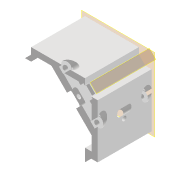
# Autodesk Inventor part: 20_Cube_Insert_Kinematic_Mirror_45_pro_v3
Saved by Autodesk Inventor 2022 (Build 260153000, 153)
## iProperties
Created: 2022-01-05
Part Number: 20_Cube_Insert_Kinematic_Mirror_45_pro_v3
Material: Generisch
Document SubType Name: Modeling
Designer: diederichbenedict
Density: 1 g/cm^3
Appearance: Vorgabe
Author: diederichbenedict
Autodesk Inventor part; units mm, degrees
ref_plane "YZ Plane" through (0, 0, 0) normal (1, 0, 0) x (0, 1, 0)
ref_plane "XZ Plane" through (0, 0, 0) normal (0, 1, 0) x (-1, 0, 0)
ref_plane "XY Plane" through (0, 0, 0) normal (0, 0, 1) x (1, 0, 0)
ref_plane "Arbeitsebene1" through (0, 0, 0) normal (0, 0, 1) x (1, 0, 0)
sketch "Skizze1" plane through (0, 0, 0) normal (0, 0, 1) x (1, 0, 0)
  arc A0 (24.85, 22.85) -> (22.85, 24.85) centre (22.85, 22.85) ccw projected
  line L0 (22.85, 24.85) -> (-16.97, 24.85) projected
  line L1 (-16.97, 24.85) -> (-16.97, 21.15) projected
  line L2 (-16.97, 21.15) -> (16.97, 21.15) projected
  line L3 (16.97, 16.97) -> (16.97, 21.15) projected
  line L4 (21.15, 16.97) -> (16.97, 16.97) projected
  line L5 (21.15, 16.97) -> (21.15, -16.97) projected
  line L6 (21.15, -16.97) -> (24.85, -16.97) projected
  line L7 (24.85, -16.97) -> (24.85, 22.85) projected
  line L8 (23.75, 23.25) -> (23.75, 18.15) projected
  arc A1 (23.25, 17.65) -> (23.75, 18.15) centre (23.25, 18.15) ccw projected
  line L9 (23.25, 17.65) -> (20.8937, 17.65) projected
  arc A2 (20.5239, 17.8134) -> (20.8937, 17.65) centre (20.8937, 18.15) ccw projected
  line L10 (20.5239, 17.8134) -> (17.7803, 20.8273) projected
  arc A3 (17.65, 21.1639) -> (17.7803, 20.8273) centre (18.15, 21.1639) ccw projected
  line L11 (17.65, 21.1639) -> (17.65, 23.25) projected
  arc A4 (18.15, 23.75) -> (17.65, 23.25) centre (18.15, 23.25) ccw projected
  line L12 (18.15, 23.75) -> (23.25, 23.75) projected
  arc A5 (23.75, 23.25) -> (23.25, 23.75) centre (23.25, 23.25) ccw projected
  line L13 (-16.87, 24.85) -> (16.87, 24.85)
  line L14 (16.87, 24.85) -> (16.87, 21.85)
  line L15 (16.87, 21.85) -> (-16.87, 21.85)
  line L16 (-16.87, 21.85) -> (-16.87, 24.85)
  line L17 (34.79, 34.79) -> (-34.79, -34.79)
  line L18 (16.87, 21.85) -> (16.87, 16.87)
  line L19 (12.87, 21.85) -> (12.87, 12.87)
  line L20 (16.87, 16.87) -> (12.87, 12.87)
  line L21 (-16.97, 21.15) -> (-16.97, 16.97) projected
  line L22 (16.97, 16.97) -> (-16.97, 16.97) projected
  line L23 (16.97, 21.15) -> (16.97, 16.97) projected
  line L24 (-16.97, 21.15) -> (16.97, 21.15) projected
  line L25 (-16.97, 16.97) -> (-16.97, 20.75) projected
  line L26 (-20.75, 16.97) -> (-16.97, 20.75) projected
  line L27 (-20.75, 16.97) -> (-16.97, 16.97) projected
  line L28 (-16.87, 21.85) -> (-12.87, 21.85)
  line L29 (-12.87, 21.85) -> (-12.87, 16.97)
  line L30 (-12.87, 16.97) -> (-16.87, 16.97)
  line L31 (-16.87, 16.97) -> (-16.87, 21.85)
  line L32 (-16.87, 20.7793) -> (-20.6793, 16.97)
  line L33 (-20.6793, 16.97) -> (-16.87, 16.97)
  line L34 (-4.8794, 21.85) -> (21.15, -4.1794)
  line L35 (-7.0711, 15.5563) -> (3.471, 5.0143) projected
  line L36 (21.15, 2.8916) -> (2.1916, 21.85)
  line L37 (12.0208, 12.0208) -> (8.4853, 8.4853)
  line L38 (20.75, 16.97) -> (16.97, 20.75) projected
  line L39 (16.97, 20.6793) -> (20.6793, 16.97)
  point P0 (0, 0)
  point P1 (-12.87, 21.15)
  point P2 (12.87, 21.15)
  point P3 (2.8916, 21.15)
  point P4 (-4.1794, 21.15)
  point P5 (12.87, 16.97)
  point P6 (16.87, 21.15)
  dimension "d0" = 0.1
  dimension "d1" = 0.1
  dimension "d2" = 3
  dimension "d3" = 4
  dimension "d6" = 4
  dimension "d8" = 0
  dimension "d9" = 0.05
  dimension "d10" = 6
  dimension "d11" = 5
  dimension "d12" = 0.05
  constraints: 36 end point, 16 point on line, 8 parallel, 2 horizontal, 2 perpendicular, 1 collinear, 1 vertical, 3 other
  measures "d0" distance between parallel lines of L16 L1
  measures "d1" distance between parallel lines of L14 L3
  measures "d2" distance between parallel lines of L0 L15
  measures "d3" distance between parallel lines of L18 L19
  measures "d6" distance of L29.end L30.end
  measures "d8" distance between parallel lines of L30 L22
  measures "d9" distance between parallel lines of L26 L32
  measures "d10" distance between parallel lines of L35 L34
  measures "d11" distance between parallel lines of L36 L34
  measures "d12" distance between parallel lines of L39 L38
extrude "Extrusion1" add sketch "Skizze1" along normal blind 33.8 contours L14 L15 L16 L0 | L18 L2 L19 L15 | L34 L22 L36 L17 | L15 L29 L2 L31 | L19 L2 L36 L15 | L18 L22 L19 L2 | L2 L3 L22 L18 | L39 L4 L17 | L17 L3 L39 | L34 L2 L36 L22 | L15 L34 L2 L29 | L2 L29 L22 L31 | L36 L2 L34 L15 | L31 L22 L21 L32 | L21 L27 L32
mirror "Spiegeln1" about plane through (8.4853, 8.4853, 0) normal (0.7071, -0.7071, 0) of "Extrusion1"
chamfer "Fase1" distance 4 angle 45 3 edges at (12.87, 16.97, 16.9) (16.97, 12.87, 16.9) (-12.87, 16.97, 16.9)
ref_plane "Arbeitsebene2" through (21.9197, 25.629, 0) normal (0.7071, 0.7071, 0) x (-0.7071, 0.7071, 0)
sketch "Skizze2" plane through (21.9197, 25.629, 0) normal (0.7071, 0.7071, 0) x (-0.7071, 0.7071, 0)
  line L0 (-16.6229, 20.13) -> (-16.6229, 14.13) projected
  arc A0 (-19.6229, 14.13) -> (-16.6229, 14.13) centre (-18.1229, 14.13) ccw projected
  line L1 (-19.6229, 14.13) -> (-19.6229, 20.13) projected
  arc A1 (-16.6229, 20.13) -> (-19.6229, 20.13) centre (-18.1229, 20.13) ccw projected
  line L2 (0.3771, 31.21) -> (-5.6229, 31.21) projected
  arc A2 (-5.6229, 34.21) -> (-5.6229, 31.21) centre (-5.6229, 32.71) ccw projected
  line L3 (-5.6229, 34.21) -> (0.3771, 34.21) projected
  arc A3 (0.3771, 31.21) -> (0.3771, 34.21) centre (0.3771, 32.71) ccw projected
  circle A4 centre (-16.6229, 31.13) radius 3.25 projected
  circle A5 centre (-2.6229, 17.13) radius 3.25 projected
  circle A6 centre (11.3771, 31.13) radius 3.25 projected
  circle A7 centre (-16.6229, 3.13) radius 3.25 projected
  line L4 (14.3357, 42.03) -> (-19.6229, 42.03) projected
  line L5 (-19.6229, 42.03) -> (-19.6229, 38.4552) projected
  line L6 (-19.6229, 38.4552) -> (-23.9481, 34.13) projected
  line L7 (-23.9481, 34.13) -> (-27.5229, 34.13) projected
  line L8 (-27.5229, 34.13) -> (-27.5229, 0.13) projected
  line L9 (-27.5229, 0.13) -> (-23.9481, 0.13) projected
  line L10 (-23.9481, 0.13) -> (-19.6229, -4.1952) projected
  line L11 (-19.6229, -4.1952) -> (-19.6229, -7.77) projected
  line L12 (-19.6229, -7.77) -> (14.3771, -7.77) projected
  line L13 (14.3771, -7.77) -> (14.3771, -4.1952) projected
  line L14 (14.3771, -4.1952) -> (18.7023, 0.13) projected
  line L15 (18.7023, 0.13) -> (22.2771, 0.13) projected
  line L16 (22.2771, 0.13) -> (22.2771, 34.13) projected
  line L17 (22.2771, 34.13) -> (18.7023, 34.13) projected
  line L18 (18.7023, 34.13) -> (14.3357, 38.4966) projected
  line L19 (14.3357, 38.4966) -> (14.3357, 42.03) projected
  point P0 (-2.6229, 0)
hole "Bohrung1" at (13.8749, 33.6739, 31.13) at (33.6739, 13.8749, 31.13) at (33.6739, 13.8749, 3.13) direction (-0.7071, -0.7071, 0) diameter 2.8 depth 30 tip angle 118 counterbore diameter 6.5 counterbore depth 17
sketch "Skizze3" plane through (16.97, 20.6793, 0) normal (0.7071, 0.7071, 0) x (-0.7071, 0.7071, 0)
  line L0 (-16.6229, 20.13) -> (-16.6229, 14.13) projected
  arc A0 (-19.6229, 14.13) -> (-16.6229, 14.13) centre (-18.1229, 14.13) ccw projected
  line L1 (-19.6229, 14.13) -> (-19.6229, 20.13) projected
  arc A1 (-16.6229, 20.13) -> (-19.6229, 20.13) centre (-18.1229, 20.13) ccw projected
  line L2 (0.3771, 31.21) -> (-5.6229, 31.21) projected
  arc A2 (-5.6229, 34.21) -> (-5.6229, 31.21) centre (-5.6229, 32.71) ccw projected
  line L3 (-5.6229, 34.21) -> (0.3771, 34.21) projected
  arc A3 (0.3771, 31.21) -> (0.3771, 34.21) centre (0.3771, 32.71) ccw projected
  circle A4 centre (-16.6229, 31.13) radius 3.25 projected
  circle A5 centre (-2.6229, 17.13) radius 3.25 projected
  circle A6 centre (11.3771, 31.13) radius 3.25 projected
  circle A7 centre (-16.6229, 3.13) radius 3.25 projected
  line L4 (14.3357, 42.03) -> (-19.6229, 42.03) projected
  line L5 (-19.6229, 42.03) -> (-19.6229, 38.4552) projected
  line L6 (-19.6229, 38.4552) -> (-23.9481, 34.13) projected
  line L7 (-23.9481, 34.13) -> (-27.5229, 34.13) projected
  line L8 (-27.5229, 34.13) -> (-27.5229, 0.13) projected
  line L9 (-27.5229, 0.13) -> (-23.9481, 0.13) projected
  line L10 (-23.9481, 0.13) -> (-19.6229, -4.1952) projected
  line L11 (-19.6229, -4.1952) -> (-19.6229, -7.77) projected
  line L12 (-19.6229, -7.77) -> (14.3771, -7.77) projected
  line L13 (14.3771, -7.77) -> (14.3771, -4.1952) projected
  line L14 (14.3771, -4.1952) -> (18.7023, 0.13) projected
  line L15 (18.7023, 0.13) -> (22.2771, 0.13) projected
  line L16 (22.2771, 0.13) -> (22.2771, 34.13) projected
  line L17 (22.2771, 34.13) -> (18.7023, 34.13) projected
  line L18 (18.7023, 34.13) -> (14.3357, 38.4966) projected
  line L19 (14.3357, 38.4966) -> (14.3357, 42.03) projected
  point P0 (-2.6229, 0)
extrude "Extrusion2" cut sketch "Skizze3" against normal blind 33.8 contours L0 A0 L1 A1 | L2 A2 L3 A3
sketch "Skizze4" plane through (0, 0, 33.8) normal (0, 0, 1) x (1, 0, 0)
  line L0 (10.6066, 6.364) -> (6.364, 10.6066) projected
  line L1 (14.1421, 9.8995) -> (10.6066, 6.364) projected
  line L2 (9.8995, 14.1421) -> (14.1421, 9.8995) projected
  line L3 (9.8995, 14.1421) -> (6.364, 10.6066) projected
  circle A0 centre (10.3701, 10.3701) radius 1.4
  point P0 (0, 0)
  dimension "d26" = 2.8
  constraints: 1 centre point
  measures "d26" diameter of A0
extrude "Extrusion3" cut sketch "Skizze4" against normal blind 20 contours A0
sketch "Skizze5" plane through (24.85, -16.87, 33.8) normal (1, 0, 0) x (0, 0, -1)
  ellipse E0 centre (13.67, 19.7997) end of major axis (13.67, 21.921) minor radius 1.5 (13.67, 21.921) -> (13.67, 17.6784) ccw projected
  line L0 (13.67, 21.921) -> (19.67, 21.921) projected
  ellipse E1 centre (19.67, 19.7997) end of major axis (19.67, 17.6784) minor radius 1.5 (19.67, 17.6784) -> (19.67, 21.921) ccw projected
  line L1 (19.67, 17.6784) -> (13.67, 17.6784) projected
  ellipse E2 centre (2.67, 21.921) end of major axis (2.67, 26.5172) minor radius 3.25 (0, 19.3005) -> (0, 24.5415) ccw projected
  line L2 (0, 19.3005) -> (0, 0) projected
  line L3 (33.8, 0) -> (0, 0) projected
  line L4 (33.8, 20.6836) -> (33.8, 0) projected
  ellipse E3 centre (30.67, 21.921) end of major axis (30.67, 26.5172) minor radius 3.25 (33.8, 23.1584) -> (33.8, 20.6836) ccw projected
  line L5 (33.8, 33.74) -> (33.8, 23.1584) projected
  line L6 (33.8, 33.74) -> (0, 33.74) projected
  line L7 (0, 33.74) -> (0, 24.5415) projected
  line L8 (19.67, 15.4558) -> (13.67, 15.4558) projected
  circle A0 centre (16.67, 15.4558) radius 1.4
  point P0 (33.8, 16.87)
  dimension "d29" = 2.8
  constraints: 1 centre point, 1 midpoint, 4 other
  measures "d29" diameter of A0
extrude "Extrusion4" cut sketch "Skizze5" against normal blind 20 contours A0 L8 | L8 A0
